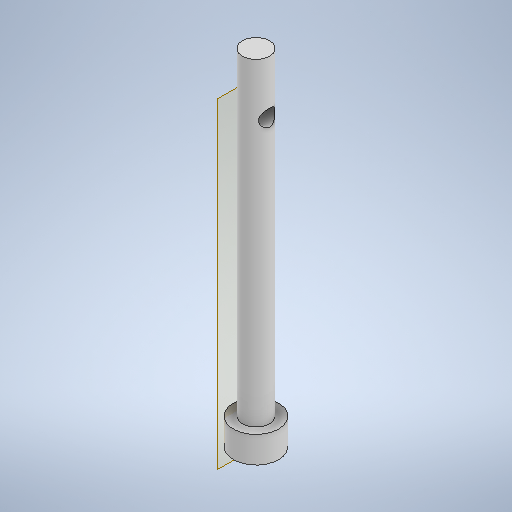
# Autodesk Inventor part: sworzen
Saved by Autodesk Inventor 2025.2 (Build 292293000, 293)
## iProperties
Created: 2025-11-27
Part Number: sworzen
Material: Ogólny
Document SubType Name: Modeling
Designer: juras
Density: 1 g/cm^3
Appearance: Domyślna
Author: juras
Autodesk Inventor part; units mm, degrees
ref_plane "XZ Plane" through (0, 0, 0) normal (0, 1, 0) x (-1, 0, 0)
ref_plane "XY Plane" through (0, 0, 0) normal (0, 0, 1) x (1, 0, 0)
sketch "Szkic1" plane through (0, 0, 0) normal (0, 1, 0) x (-1, 0, 0)
  circle A0 centre (0, 0) radius 4.25
  dimension "d0" = 8.5
  constraints: 1 centre point, 1 coincident
  measures "d0" diameter of A0
extrude "Wyciągnięcie proste1" add sketch "Szkic1" along normal mid plane 5
sketch "Szkic2" plane through (0, 2.5, 0) normal (0, 1, 0) x (1, 0, 0)
  circle A0 centre (0, 0) radius 2.55
  dimension "d3" = 5.1
  constraints: 1 centre point, 1 coincident
  measures "d3" diameter of A0
extrude "Wyciągnięcie proste2" add sketch "Szkic2" along normal blind 60
ref_plane "Płaszczyzna konstrukcyjna1" through (-2.65, 0, 0) normal (1, 0, 0) x (0, 1, 0)
sketch "Szkic3" plane through (-2.65, 0, 0) normal (1, 0, 0) x (0, 1, 0)
  point P0 (0, 0)
sketch "Szkic4" plane through (-2.65, 0, 0) normal (1, 0, 0) x (0, 1, 0)
  circle A0 centre (52.5, 0) radius 1.55
  line L0 (62.5, -2.55) -> (62.5, 2.55) projected
  point P0 (0, 0)
  dimension "d8" = 3.1
  dimension "d9" = 10
  constraints: 1 centre point
  measures "d8" diameter of A0
  measures "d9" distance from line of L0 A0.centre
extrude "Wyciągnięcie proste3" cut sketch "Szkic4" along normal blind 50
